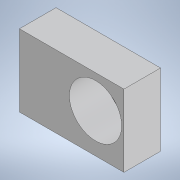
# Autodesk Inventor part: Screen_Spacers
Saved by Autodesk Inventor 2020 (Build 240168000, 168)
## iProperties
Created: 2021-11-22
Part Number: Screen_Spacers
Material: Generic
Document SubType Name: Modeling
Designer: mtkts
Density: 1 g/cm^3
Appearance: Default
Author: mtkts
Autodesk Inventor part; units mm, degrees
ref_plane "YZ Plane" through (0, 0, 0) normal (1, 0, 0) x (0, 1, 0)
ref_plane "XZ Plane" through (0, 0, 0) normal (0, 1, 0) x (-1, 0, 0)
ref_plane "XY Plane" through (0, 0, 0) normal (0, 0, 1) x (1, 0, 0)
sketch "Sketch1" plane through (0, 0, 0) normal (0, 0, 1) x (1, 0, 0)
  circle A0 centre (47.5, 66.25) radius 1.5 projected
  line L0 (50.22, 62.5) -> (-50.22, 62.5) construction
  line L1 (50.22, 62.5) -> (50.22, 69.4) construction
  line L2 (50.22, 69.4) -> (-50.22, 69.4) construction
  line L3 (50.22, 69.4) -> (40.22, 69.4)
  line L4 (40.22, 69.4) -> (40.22, 62.5)
  line L5 (40.22, 62.5) -> (50.22, 62.5)
  line L6 (50.22, 62.5) -> (50.22, 69.4)
  point P0 (0, 0)
  dimension "d0" = 10
  constraints: 8 end point, 2 parallel, 1 horizontal, 1 perpendicular, 1 point on line
  measures "d0" distance of L5.end L4.end
extrude "Extrusion1" add sketch "Sketch1" along normal blind 3.5
sketch "Sketch2" plane through (0, 0, 3.5) normal (0, 0, 1) x (1, 0, 0)
  circle A0 centre (47.5, 66.25) radius 1.5 projected
  circle A1 centre (47.5, 66.25) radius 2.5
  point P0 (0, 0)
  dimension "d3" = 1
  constraints: 1 centre point
  measures "d3" radial gap between concentric circles of A0 A1
extrude "Extrusion2" cut sketch "Sketch2" against normal through all
body "Solid1"
